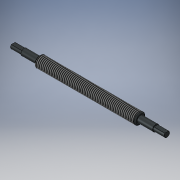
# Autodesk Inventor part: КВ33.000.104 - Вал
Saved by Autodesk Inventor 2019 (Build 230136000, 136)
## iProperties
Created: 2021-04-18
Part Number: КВ33.000.104 - Вал
Material: Iron, Ductile
Document SubType Name: Modeling
Designer: Петров Иван
Density: 7.15 g/cm^3
Appearance: Iron Gray
Author: Петров Иван
Autodesk Inventor part; units mm, degrees
ref_plane "YZ Plane" through (0, 0, 0) normal (1, 0, 0) x (0, 1, 0)
ref_plane "XZ Plane" through (0, 0, 0) normal (0, 1, 0) x (-1, 0, 0)
ref_plane "XY Plane" through (0, 0, 0) normal (0, 0, 1) x (1, 0, 0)
sketch "Sketch1" plane through (0, 0, 0) normal (1, 0, 0) x (0, 1, 0)
  circle A0 centre (0, 0) radius 5
  dimension "d0" = 10
  constraints: 1 centre point, 1 coincident
  measures "d0" diameter of A0
extrude "Extrusion1" add sketch "Sketch1" along normal blind 46
thread "Thread1" size "M10x1.5" class "6g" standard "ANSI Metric M Profile" full length
chamfer "Chamfer1" distance 1 angle 45 1 edges at (46, -5, 0)
sketch "Sketch2" plane through (46, 0, 0) normal (1, 0, 0) x (0, 0, -1)
  circle A0 centre (0, 0) radius 3
  dimension "d8" = 6
  constraints: 1 centre point, 1 coincident
  measures "d8" diameter of A0
extrude "Extrusion2" add sketch "Sketch2" along normal blind 14
sketch "Sketch3" plane through (60, 0, 0) normal (1, 0, 0) x (0, 0, -1)
  circle A0 centre (0, 0) radius 2.5
  line L0 (-1.7349, 1.8) -> (1.7349, 1.8)
  dimension "d11" = 5
  dimension "d12" = 1.8
  constraints: 2 end point, 2 point on circle, 1 centre point, 1 coincident, 1 horizontal
  measures "d11" diameter of A0
  measures "d12" distance from line of point (0, 0) L0
extrude "Extrusion3" add sketch "Sketch3" along normal blind 10 contours A0 L0 picked at (0.076, 0.3701)
mirror "Mirror1" about plane through (0, 0, 0) normal (-1, 0, 0) of "Extrusion1", "Chamfer1", "Extrusion2", "Extrusion3"
body "Solid1"
